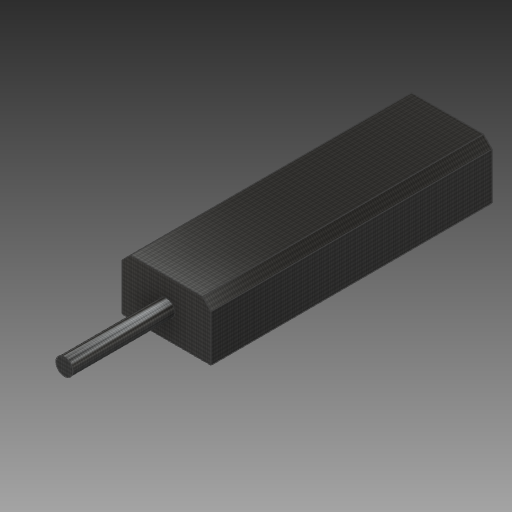
# Autodesk Inventor part: chineese z
Saved by Autodesk Inventor 2019 (Build 230136000, 136)
## iProperties
Created: 2017-12-22
Part Number: chineese z
Material: Generic
Document SubType Name: Modeling
Designer: torba
Density: 1 g/cm^3
Appearance: Engine Turned
Author: torba
Autodesk Inventor part; units mm, degrees
ref_plane "YZ Plane" through (0, 0, 0) normal (1, 0, 0) x (0, 1, 0)
ref_plane "XZ Plane" through (0, 0, 0) normal (0, 1, 0) x (-1, 0, 0)
ref_plane "XY Plane" through (0, 0, 0) normal (0, 0, 1) x (1, 0, 0)
sketch "Sketch1" plane through (0, 0, 0) normal (0, 1, 0) x (-1, 0, 0)
  line L0 (0, 0) -> (131, 0)
  line L1 (131, 0) -> (131, -413)
  line L2 (131, -413) -> (0, -413)
  line L3 (0, -413) -> (0, 0)
  dimension "d0" = 131
  dimension "d1" = 413
  constraints: 8 end point, 2 parallel, 1 horizontal, 1 perpendicular
  measures "d0" distance of L1.end L2.end
  measures "d1" distance of L0.end L1.end
extrude "Extrusion1" add sketch "Sketch1" along normal blind 81
sketch "Sketch2" plane through (-131, 0, 0) normal (0, 0, 1) x (1, 0, 0)
  line L0 (131, 0) -> (0, 0) projected
  line L1 (131, 0) -> (131, 81) projected
  line L2 (0, 81) -> (131, 81) projected
  line L3 (0, 0) -> (0, 81) projected
  line L4 (0, 81) -> (131, 0) construction
  circle A0 centre (65.5, 40.5) radius 12.5
  dimension "d4" = 25
  constraints: 2 end point, 1 centre point, 1 midpoint
  measures "d4" diameter of A0
extrude "Extrusion2" add sketch "Sketch2" along normal blind 150 contours A0
sketch "Sketch3" plane through (0, 0, 0) normal (0, -1, 0) x (1, 0, 0)
  line L0 (0, 0) -> (-131, 0) projected
  line L1 (-131, 0) -> (-131, -413) projected
  line L2 (-131, -413) -> (0, -413) projected
  line L3 (0, -413) -> (0, 0) projected
  line L4 (0, -413) -> (-131, -413) projected
  line L5 (-65.5, -413) -> (-65.5, 0) construction
  line L6 (-131, 0) -> (0, 0) projected
  line L7 (-65.5, -70) -> (-98.5, -70)
  line L8 (-65.5, -483) -> (-65.5, -70) construction
  line L9 (-65.5, -553) -> (-65.5, -140) construction
  line L10 (0.5, -413) -> (0.5, 0) construction
  line L11 (0.5, -483) -> (0.5, -70) construction
  line L12 (0.5, -553) -> (0.5, -140) construction
  point P0 (-65.5, -140)
  point P1 (-98.5, -140)
  point P2 (-65.5, -210)
  point P3 (-98.5, -210)
  point P4 (0.5, -70)
  point P5 (-32.5, -70)
  point P6 (0.5, -140)
  point P7 (-32.5, -140)
  point P8 (0.5, -210)
  point P9 (-32.5, -210)
  dimension "d7" = 33
  dimension "d10" = 70
  dimension "d13" = 66
  dimension "d16" = 70
  constraints: 14 end point, 6 point on line, 2 horizontal, 2 midpoint, 1 coincident, 1 vertical, 25 other
  measures "d7" distance of L7.start L7.end
  measures "d10" distance of L5.start L8.start
  measures "d13" distance of L5.start L10.start
  measures "d16" distance between parallel lines of L0 L7
hole "Hole1" at (-98.5, 0, -70) at (-98.5, 0, -140) at (-98.5, 0, -210) at (-32.5, 0, -70) at (-32.5, 0, -140) at (-32.5, 0, -210) direction (0, 1, 0) diameter 5 depth 25.4 tip angle 118
chamfer "Chamfer1" distance 12.7 angle 45 2 edges at (0, 81, -206.5) (-131, 81, -206.5)
body "Solid1"
